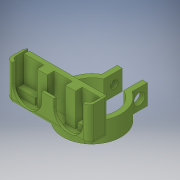
# Autodesk Inventor part: Ultrasonic Mount 1.14in
Saved by Autodesk Inventor 2018 (Build 220112000, 112)
## iProperties
Created: 2018-01-09
Part Number: Ultrasonic Mount 1.14in
Material: PC/ABS Plastic
Document SubType Name: Modeling
Designer: prakh
Density: 0.357273 g/cm^3
Appearance: Olive Green
Author: prakh
Autodesk Inventor part; units mm, degrees
ref_plane "YZ Plane" through (0, 0, 0) normal (1, 0, 0) x (0, 1, 0)
ref_plane "XZ Plane" through (0, 0, 0) normal (0, 1, 0) x (-1, 0, 0)
ref_plane "XY Plane" through (0, 0, 0) normal (0, 0, 1) x (1, 0, 0)
sketch "Sketch1" plane through (0, 0, 0) normal (0, 0, 1) x (1, 0, 0)
  arc A0 (13.7142, 6.35) -> (13.7142, -6.35) centre (0, 0) ccw
  line L0 (25.4, -9.525) -> (15.6117, -9.525)
  line L1 (6.1638, -4.445) -> (6.1638, -1.27)
  line L2 (13.7142, -6.35) -> (25.4, -6.35)
  line L3 (25.4, -6.35) -> (25.4, -9.525)
  line L4 (25.4, 6.35) -> (13.7142, 6.35)
  line L5 (8.3094, 1.6345) -> (8.3094, 4.8095)
  line L6 (25.4, 9.525) -> (25.4, 6.35)
  line L7 (15.6117, 9.525) -> (25.4, 9.525)
  arc A1 (15.6117, 9.525) -> (15.6117, -9.525) centre (0, 0) ccw
  dimension "d0" = 30.226
  dimension "d2" = 3.175
  dimension "d3" = 9.525
  dimension "d4" = 25.4
  dimension "d5" = 3.175
  constraints: 16 end point, 4 parallel, 4 point on circle, 2 centre point, 2 coincident, 2 equal length, 2 horizontal, 2 perpendicular, 1 collinear
  measures "d0" diameter of A0
  measures "d2" distance of L2.end L0.start
  measures "d3" distance from line of point (0, 0) L0
  measures "d4" distance from line of point (0, 0) L3
  measures "d5" radial gap between concentric circles of A0 A1
extrude "Extrusion1" add sketch "Sketch1" along normal blind 12.7
sketch "Sketch2" plane through (15.6117, 9.525, 0) normal (0, 1, 0) x (1, 0, 0)
  circle A0 centre (4.7083, -6.35) radius 2.4638
  line L0 (9.7883, -12.7) -> (0, -12.7) projected
  line L1 (9.7883, 0) -> (9.7883, -12.7) projected
  point P0 (-15.6117, 0)
  dimension "d8" = 6.35
  dimension "d9" = 5.08
  dimension "d10" = 4.9276
  constraints: 1 centre point
  measures "d8" distance from line of A0.centre L0
  measures "d9" distance from line of A0.centre L1
  measures "d10" diameter of A0
extrude "Extrusion2" cut sketch "Sketch2" against normal blind 25.4
sketch "Sketch3" plane through (15.6117, 9.525, 0) normal (0, 1, 0) x (1, 0, 0)
  circle A0 centre (4.7083, -6.35) radius 2.4638 projected
  circle A1 centre (4.7083, -6.35) radius 3.4798
  point P0 (-15.6117, 0)
  dimension "d13" = 1.016
  constraints: 1 centre point, 1 coincident
  measures "d13" radial gap between concentric circles of A0 A1
extrude "Extrusion3" cut sketch "Sketch3" against normal up to surface (3.175 mm away)
sketch "Sketch4" plane through (0, 0, 0) normal (0, 0, -1) x (-1, 0, 0)
  line L0 (18.288, -24.765) -> (15.113, -24.765)
  line L1 (15.113, -24.765) -> (15.113, 24.765)
  line L2 (15.113, 24.765) -> (18.288, 24.765)
  line L3 (18.288, 24.765) -> (18.288, -24.765)
  arc A0 (-13.7142, -6.35) -> (-13.7142, 6.35) centre (0, 0) ccw projected
  arc A1 (-15.6117, -9.525) -> (-15.6117, 9.525) centre (0, 0) ccw projected
  dimension "d20" = 49.53
  dimension "d21" = 24.765
  constraints: 8 end point, 2 parallel, 2 tangent, 1 horizontal, 1 perpendicular
  measures "d20" distance between parallel lines of L0 L2
  measures "d21" distance from line of point (0, 0) L0
extrude "Extrusion4" add sketch "Sketch4" along normal blind 20.6375
sketch "Sketch5" plane through (-15.113, -24.765, 0) normal (1, 0, 0) x (0, 0, -1)
  line L0 (21.9075, -1.27) -> (-1.27, -1.27)
  line L1 (-1.27, 50.8) -> (21.9075, 50.8)
  line L2 (0, 49.53) -> (20.6375, 49.53) projected
  line L3 (0, 35.063) -> (0, 49.53) projected
  line L4 (0, 0) -> (20.6375, 0) projected
  line L5 (20.6375, 0) -> (0, 0)
  line L6 (0, 49.53) -> (20.6375, 49.53)
  line L7 (20.6375, 49.53) -> (21.9075, 49.53)
  line L8 (20.6375, 0) -> (21.9075, 0)
  line L9 (0, 30.48) -> (-1.27, 30.48)
  line L10 (0, 19.05) -> (-1.27, 19.05)
  line L11 (21.9075, 50.8) -> (21.9075, 49.53)
  line L12 (21.9075, 0) -> (21.9075, -1.27)
  line L13 (-1.27, -1.27) -> (-1.27, 19.05)
  line L14 (-1.27, 30.48) -> (-1.27, 50.8)
  line L15 (0, 0) -> (0, 19.05)
  line L16 (0, 30.48) -> (0, 49.53)
  point P0 (0, 24.765)
  dimension "d22" = 1.27
  dimension "d24" = 1.27
  dimension "d28" = 23.1775
  dimension "d29" = 20.32
  dimension "d30" = 1.27
  dimension "d31" = 1.27
  constraints: 28 end point, 6 horizontal, 6 parallel, 4 perpendicular, 2 equal length, 1 collinear
  measures "d22" distance between parallel lines of L1 L2
  measures "d24" distance between parallel lines of L0 L4
  measures "d28" distance of L1.start L1.end
  measures "d29" distance of L9.end L1.start
  measures "d30" distance between parallel lines of L3 L14
  measures "d31" distance between parallel lines of L15 L13
extrude "Extrusion5" add sketch "Sketch5" against normal blind 11.303
sketch "Sketch7" plane through (-18.288, -5.715, 0) normal (-1, 0, 0) x (0, 0, 1)
  line L0 (0, 30.48) -> (0, 11.43) projected
  line L1 (0, 30.48) -> (-20.6375, 30.48) projected
  line L2 (-20.6375, -19.05) -> (-20.6375, 30.48) projected
  line L3 (0, -19.05) -> (-20.6375, -19.05) projected
  line L4 (0, 0) -> (0, -19.05) projected
  line L5 (0, 5.715) -> (0, 0) projected
  line L6 (0, 11.43) -> (0, 5.715) projected
  line L7 (0, -19.05) -> (-4.114, -19.05)
  line L8 (-4.114, -19.05) -> (-4.114, -7.62)
  line L9 (-4.114, -7.62) -> (0, -7.62)
  line L10 (0, -7.62) -> (0, -19.05)
  line L11 (0, 30.48) -> (-4.114, 30.48)
  line L12 (-4.114, 30.48) -> (-4.114, 19.05)
  line L13 (-4.114, 19.05) -> (0, 19.05)
  line L14 (0, 19.05) -> (0, 30.48)
  point P0 (0, 5.715)
  constraints: 16 end point, 4 parallel, 2 horizontal, 2 perpendicular, 1 point on line
extrude "Extrusion7" add sketch "Sketch7" along normal blind 4.318 contours L0 L13 L12 L1 | L8 L9 L4 L3
sketch "Sketch8" plane through (-18.288, -13.335, 0) normal (-1, 0, 0) x (0, 0, 1)
  line L0 (0, 13.335) -> (0, 7.62) projected
  line L1 (0, 1.27) -> (-20.6375, 1.27)
  line L2 (-20.6375, 1.27) -> (-20.6375, 7.62)
  line L3 (-20.6375, 7.62) -> (0, 7.62)
  line L4 (0, 7.62) -> (0, 1.27)
  line L5 (-20.6375, 19.05) -> (0, 19.05)
  line L6 (0, 19.05) -> (0, 25.4)
  line L7 (0, 25.4) -> (-20.6375, 25.4)
  line L8 (-20.6375, 25.4) -> (-20.6375, 19.05)
  line L9 (-20.6375, -11.43) -> (-20.6375, 38.1) projected
  line L10 (-21.9075, 38.1) -> (0, 38.1) projected
  line L11 (0, -11.43) -> (-21.9075, -11.43) projected
  point P0 (0, 0)
  dimension "d37" = 6.35
  dimension "d38" = 6.35
  dimension "d39" = 12.7
  dimension "d40" = 12.7
  constraints: 16 end point, 4 parallel, 3 point on line, 2 horizontal, 2 perpendicular, 1 collinear
  measures "d37" distance between parallel lines of L5 L7
  measures "d38" distance of L1.end L2.end
  measures "d39" distance between parallel lines of L7 L10
  measures "d40" distance between parallel lines of L1 L11
extrude "Extrusion8" add sketch "Sketch8" along normal up to surface (4.318 mm away)
sketch "Sketch9" plane through (-26.416, -24.765, 0) normal (-1, 0, 0) x (0, 0, 1)
  line L0 (1.27, -1.27) -> (1.27, 14.467) projected
  line L1 (1.27, 50.8) -> (-21.9075, 50.8) projected
  line L2 (1.27, -1.27) -> (-21.9075, -1.27)
  line L3 (-21.9075, 50.8) -> (1.27, 50.8)
  line L4 (1.27, 50.8) -> (1.27, -1.27)
  circle A0 centre (-9.9999, 11.7693) radius 8.0001 projected
  circle A1 centre (-10.0001, 37.7692) radius 7.9998 projected
  arc A2 (-9.9999, 2.4992) -> (-9.9999, 21.0394) centre (-9.9999, 11.7693) ccw
  arc A3 (-10.0001, 28.4994) -> (-10.0001, 47.0391) centre (-10.0001, 37.7692) ccw
  line L5 (-10.0001, 47.0391) -> (-21.9075, 47.0391)
  line L6 (-10.0001, 28.4994) -> (-15.11, 28.4994)
  line L7 (-9.9999, 21.0394) -> (-15.11, 21.0394)
  line L8 (-9.9999, 2.4992) -> (-21.9075, 2.4992)
  line L9 (-21.9075, -1.27) -> (-21.9075, 2.4992)
  line L10 (-15.11, 21.0394) -> (-15.11, 28.4994)
  line L11 (-21.9075, 47.0391) -> (-21.9075, 50.8)
  line L12 (-16.38, 21.2694) -> (-16.38, 28.2694) projected
  point P0 (0, 24.765)
  point P1 (1.27, 11.43)
  dimension "d43" = 1.27
  dimension "d44" = 1.27
  dimension "d47" = 1.27
  constraints: 20 end point, 15 perpendicular, 4 parallel, 4 point on circle, 4 tangent, 2 centre point, 2 coincident, 1 collinear, 1 horizontal
  measures "d43" radial gap between concentric circles of A3 A1
  measures "d44" radial gap between concentric circles of A2 A0
  measures "d47" distance between parallel lines of L10 L12
extrude "Extrusion9" add sketch "Sketch9" along normal blind 1.5875 contours L2 L9 L8 A2 L7 L10 L6 A3 L5 L11 L1 L4 L0
fillet "Fillet1" radius 3.175 9 edges at (-21.5583, -26.035, 1.27) (-21.5582, 26.035, 1.27) (-28.0035, 0, 1.27) (-28.0035, 26.035, -10.3187) (-28.0035, -26.035, -10.3187) (-15.113, -26.035, -10.3188) (-15.113, 26.035, -10.3187) (-26.416, 24.765, -10.9537) (-26.416, -24.765, -10.9538)
fillet "Fillet2" radius 6.35 4 edges at (-16.4034, 8.0858, 1.27) (-16.4034, -8.0858, 1.27) (-15.113, 5.149, 0) (-15.113, -5.149, 0)
fillet "Fillet3" radius 3.175 2 edges at (-15.113, 10.298, 0.635) (-15.113, -10.298, 0.635)
equation "\"d21\" = 0.5 * d20"
equation "\"d24\" = d22"
equation "\"d30\" = d22"
equation "\"d31\" = d22"
equation "\"d38\" = d37"
equation "\"d40\" = d39"
equation "\"d44\" = d43"
equation "\"d23\" = d22"
equation "\"d25\" = d22"
body "Solid1"
